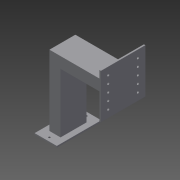
# Autodesk Inventor part: Mount
Saved by Autodesk Inventor 2013 SP1 (Build 170176100, 176)
## iProperties
Created: 2013-03-29
Part Number: Mount
Material: Generic
Document SubType Name: Modeling
Designer: tyler.camp
Density: 1 g/cm^3
Author: tyler.camp
Autodesk Inventor part; units mm, degrees
ref_plane "YZ Plane" through (0, 0, 0) normal (1, 0, 0) x (0, 1, 0)
ref_plane "XZ Plane" through (0, 0, 0) normal (0, 1, 0) x (-1, 0, 0)
ref_plane "XY Plane" through (0, 0, 0) normal (0, 0, 1) x (1, 0, 0)
sketch "Sketch1" plane through (0, 0, 0) normal (0, 1, 0) x (-1, 0, 0)
  line L0 (-38.1, 76.2) -> (38.1, 76.2)
  line L1 (38.1, 76.2) -> (38.1, -76.2)
  line L2 (38.1, -76.2) -> (-38.1, -76.2)
  line L3 (-38.1, -76.2) -> (-38.1, 76.2)
  point P0 (0, 0)
  dimension "d0" = 76.2
  dimension "d1" = 152.4
  dimension "d2" = 76.2
  dimension "d3" = 38.1
  constraints: 8 end point, 2 parallel, 1 horizontal, 1 perpendicular
  measures "d0" distance of L1.end L2.end
  measures "d1" distance of L0.end L1.end
  measures "d2" distance from line of point (0, 0) L0
  measures "d3" distance from line of point (0, 0) L3
extrude "Extrusion1" add sketch "Sketch1" along normal blind 5.08
sketch "Sketch2" plane through (0, 5.08, 0) normal (0, 1, 0) x (1, 0, 0)
  line L0 (-19.05, 44.45) -> (19.05, 44.45)
  line L1 (19.05, 44.45) -> (19.05, -44.45)
  line L2 (19.05, -44.45) -> (-19.05, -44.45)
  line L3 (-19.05, -44.45) -> (-19.05, 44.45)
  point P0 (0, 0)
  dimension "d6" = 38.1
  dimension "d7" = 88.9
  dimension "d8" = 44.45
  dimension "d9" = 19.05
  constraints: 8 end point, 2 parallel, 1 horizontal, 1 perpendicular
  measures "d6" distance of L1.end L2.end
  measures "d7" distance of L0.end L1.end
  measures "d8" distance from line of point (0, 0) L0
  measures "d9" distance from line of point (0, 0) L3
extrude "Extrusion2" add sketch "Sketch2" along normal blind 203.2
sketch "Sketch3" plane through (0, 208.28, 0) normal (0, 1, 0) x (1, 0, 0)
  line L0 (-19.05, 44.45) -> (184.15, 44.45)
  line L1 (184.15, 44.45) -> (184.15, -44.45)
  line L2 (184.15, -44.45) -> (-19.05, -44.45)
  line L3 (-19.05, -44.45) -> (-19.05, 44.45)
  line L4 (19.05, 44.45) -> (-19.05, 44.45) projected
  line L5 (-19.05, -44.45) -> (19.05, -44.45) projected
  point P0 (0, 0)
  dimension "d12" = 203.2
  constraints: 8 end point, 2 collinear, 2 parallel, 1 horizontal, 1 perpendicular
  measures "d12" distance of L1.end L2.end
extrude "Extrusion3" add sketch "Sketch3" along normal blind 38.1
sketch "Sketch4" plane through (184.15, 208.28, 44.45) normal (1, 0, 0) x (0, 0, -1)
  line L0 (-31.75, 95.25) -> (120.65, 95.25)
  line L1 (120.65, 95.25) -> (120.65, -57.15)
  line L2 (120.65, -57.15) -> (-31.75, -57.15)
  line L3 (-31.75, -57.15) -> (-31.75, 95.25)
  line L4 (0, 0) -> (88.9, 0) projected
  line L5 (88.9, 0) -> (88.9, 38.1) projected
  line L6 (0, 38.1) -> (88.9, 38.1) projected
  line L7 (0, 0) -> (0, 38.1) projected
  point P0 (44.45, -208.28)
  point P1 (44.45, 19.05)
  dimension "d20" = 76.2
  dimension "d22" = 152.4
  dimension "d23" = 76.2
  dimension "d24" = 152.4
  constraints: 8 end point, 2 parallel, 1 horizontal, 1 perpendicular, 1 other
  measures "d20" distance from line of point (44.45, 19.05) L0
  measures "d22" distance of L0.end L1.end
  measures "d23" distance from line of L3 point (44.45, 19.05)
  measures "d24" distance of L0.start L0.end
extrude "Extrusion4" add sketch "Sketch4" along normal blind 5.08 contours L0 L1 L2 L3 | L7 L6 L5 L4
sketch "Sketch5" plane through (189.23, 208.28, 44.45) normal (1, 0, 0) x (0, 0, -1)
  circle A0 centre (-6.35, 69.85) radius 3.81
  circle A1 centre (95.25, 69.85) radius 3.81
  line L0 (120.65, 95.25) -> (-31.75, 95.25) projected
  circle A2 centre (-6.35, 44.45) radius 3.81
  circle A3 centre (95.25, 44.45) radius 3.81
  circle A4 centre (-6.35, 19.05) radius 3.81
  circle A5 centre (95.25, 19.05) radius 3.81
  circle A6 centre (-6.35, -6.35) radius 3.81
  circle A7 centre (95.25, -6.35) radius 3.81
  circle A8 centre (-6.35, -31.75) radius 3.81
  circle A9 centre (95.25, -31.75) radius 3.81
  point P0 (44.45, -208.28)
  point P1 (44.45, 19.05)
  dimension "d25" = 7.62
  dimension "d27" = 152.4
  dimension "d29" = 101.6
  dimension "d30" = 50.8
  dimension "d33" = 25.4
  constraints: 10 centre point, 6 equal radius, 1 other
  measures "d25" diameter of A0
  measures "d27" distance of L0.start L0.end
  measures "d29" distance of A0.centre A1.centre
  measures "d30" horizontal distance of A0.centre point (44.45, 19.05)
  measures "d33" distance from line of L0 A1.centre
extrude "Extrusion5" cut sketch "Sketch5" against normal up to next
sketch "Sketch6" plane through (0, 5.08, 0) normal (0, 1, 0) x (1, 0, 0)
  circle A0 centre (0, 63.5) radius 3.175
  circle A1 centre (0, -63.5) radius 3.175
  line L0 (-38.1, -76.2) -> (38.1, -76.2) projected
  line L1 (38.1, 76.2) -> (-38.1, 76.2) projected
  point P0 (0, 0)
  dimension "d38" = 6.35
  dimension "d39" = 6.35
  dimension "d43" = 12.7
  dimension "d44" = 12.7
  constraints: 2 centre point
  measures "d38" diameter of A0
  measures "d39" diameter of A1
  measures "d43" distance from line of L1 A0.centre
  measures "d44" distance from line of L0 A1.centre
extrude "Extrusion6" cut sketch "Sketch6" against normal up to next
equation "\"d2\" = 0.5 * d1"
equation "\"d3\" = 0.5 * d0"
equation "\"d8\" = 0.5 * d7"
equation "\"d9\" = 0.5 * d6"
equation "\"d20\" = 0.5 * d22"
equation "\"d23\" = 0.5 * d24"
equation "\"d30\" = 0.5 * d29"
body "Solid1"
